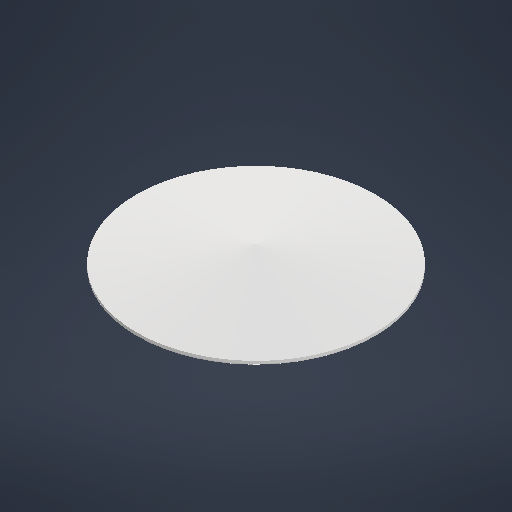
# Autodesk Inventor part: TopSpinner_steep_angle_V2
Saved by Autodesk Inventor 2026 (Build 300175050, 175E)
## iProperties
Created: 2026-04-30
Part Number: TopSpinner_steep_angle_V2
Material: Generic
Document SubType Name: Modeling
Designer: sniel
Density: 1 g/cm^3
Appearance: Default
Author: sniel
Autodesk Inventor part; units mm, degrees
ref_plane "YZ Plane" through (0, 0, 0) normal (1, 0, 0) x (0, 1, 0)
ref_plane "XZ Plane" through (0, 0, 0) normal (0, 1, 0) x (-1, 0, 0)
ref_plane "XY Plane" through (0, 0, 0) normal (0, 0, 1) x (1, 0, 0)
sketch "Sketch1" plane through (0, 0, 0) normal (1, 0, 0) x (0, 1, 0)
  line L0 (-17.6674, 93.5386) -> (-20.6674, 93.5386)
  line L1 (-20.6674, 86.1116) -> (-20.6674, 93.5386)
  line L2 (-17.6674, 86.1116) -> (-20.6674, 86.1116)
  line L3 (-17.6674, 89.9657) -> (-17.6674, 86.1116)
  arc A0 (-15.6674, 91.9657) -> (-17.6674, 89.9657) centre (-15.6674, 89.9657) ccw
  line L4 (-13.6674, 91.9657) -> (-15.6674, 91.9657)
  line L5 (-13.6674, 121.9657) -> (-13.6674, 91.9657)
  line L6 (-20.6674, 121.9657) -> (-13.6674, 121.9657)
  line L7 (-20.6674, 111.9657) -> (-20.6674, 121.9657)
  line L8 (-15.6674, 111.9657) -> (-20.6674, 111.9657)
  line L9 (-15.6674, 101.9657) -> (-15.6674, 111.9657)
  line L10 (-20.6674, 101.9657) -> (-15.6674, 101.9657)
  line L11 (-20.6674, 98.5386) -> (-20.6674, 101.9657)
  line L12 (-20.6674, 98.5386) -> (-17.6674, 98.5386)
  line L13 (-17.6674, 98.5386) -> (-17.6674, 93.5386)
  line L14 (-4.2174, -15.1948) -> (-4.2174, -7.3448)
  line L15 (-4.2174, -7.3448) -> (0.2305, -7.3448)
  circle A1 centre (-15.6674, 89.9657) radius 1.5
  line L16 (-15.6674, 91.4657) -> (-13.6674, 91.4657)
  line L17 (0.7826, -11.2698) -> (-4.2174, -11.2698)
  line L18 (0.7826, -11.2698) -> (-13.6674, 91.4657)
  line L19 (-4.2174, -7.3448) -> (-4.2174, -7.1448)
  line L20 (-4.2174, -7.1448) -> (-9.2174, -7.1448)
  line L21 (-9.2174, -7.1448) -> (-17.1624, 89.8432)
  point P0 (0, 0)
  dimension "d1" = 3
  dimension "d2" = 0.2
  dimension "d3" = 5
  constraints: 44 end point, 4 point on circle, 2 centre point, 1 coincident, 1 point on line
  measures "d1" diameter of A1
  measures "d2" distance of L14.end L19.end
  measures "d3" distance of L19.end L20.end
revolve "Revolution1" add sketch "Sketch1" angle 360 about axis through (0, 0.7826, -11.2698) along (0, -1, 0) contours L14 L15 L18 L17 | L19 L20 L21 A1 L16 L18 L15 | A1
sketch "Sketch2" plane through (0, -4.2174, -11.2698) normal (0, -1, 0) x (1, 0, 0)
  circle A0 centre (0, 0) radius 4.125 projected
  line L0 (-4.125, 0) -> (-3.125, 0)
  line L1 (-3.125, 0) -> (-3.125, -2.6926)
  line L2 (-3.125, 0) -> (-3.125, 2.6926)
  point P0 (0, 11.2698)
  dimension "d5" = 1
  constraints: 6 end point, 3 point on circle, 1 horizontal, 1 perpendicular, 1 point on line
  measures "d5" distance of L0.start L0.end
extrude "Extrusion1" add sketch "Sketch2" along normal blind 4.963 contours L2 L0 A0 | A0 L0 L1
body "Solid1"
